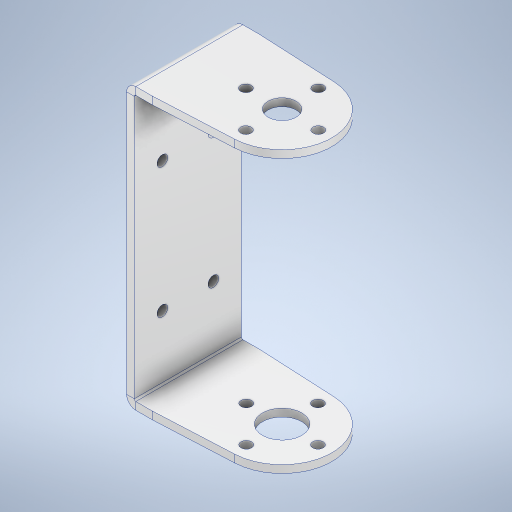
# Autodesk Inventor part: ㄷ_frame_2
Saved by Autodesk Inventor 2023 (Build 270158000, 158)
## iProperties
Created: 2022-10-22
Part Number: ㄷ_frame_2
Material: Aluminum 6061
Document SubType Name: Sheet Metal
Designer: chanh
Density: 2.7 g/cm^3
Sheet Metal Rule: Default_mm
Appearance: Aluminum - Flat
Flat Pattern Width: 2.1 cm
Flat Pattern Length: 10.9059 cm
Flat Pattern Area: 22.9023 cm^2
Sheet Metal Width: 21.000 mm
Sheet Metal Length: 109.059 mm
Sheet Metal Area: 2290.230 mm^2
품번: 20
Author: chanh
Autodesk Inventor part; units mm, degrees
ref_plane "YZ Plane" through (0, 0, 0) normal (1, 0, 0) x (0, 1, 0)
ref_plane "Work Plane1" through (34.2931, 25.9114, -33.2342) normal (0, 1, 0) x (-1, 0, 0)
sketch "Sketch2" plane through (34.2931, 25.9114, -33.2342) normal (0, 1, 0) x (-1, 0, 0)
  circle A0 centre (9.75, 7.1) radius 0.7835
  circle A1 centre (16.85, 0) radius 0.7835
  circle A2 centre (9.75, -7.1) radius 0.7835
  circle A3 centre (2.65, 0) radius 0.7835
  circle A4 centre (4.7295, -5.0205) radius 0.7835
  circle A5 centre (14.7705, -5.0205) radius 0.7835
  circle A6 centre (14.7705, 5.0205) radius 0.7835
  circle A7 centre (4.7295, 5.0205) radius 0.7835
  circle A8 centre (9.75, 0) radius 3.8
  circle A9 centre (9.75, 0) radius 9.75
  circle A10 centre (9.75, 0) radius 2.75
  line L0 (29.75, -10.5) -> (29.75, 10.5)
  line L1 (29.75, -10.5) -> (24.75, -10.5)
  line L2 (29.75, 10.5) -> (24.75, 10.5)
  line L3 (24.75, -10.5) -> (9.2707, -9.7382)
  line L4 (24.75, 10.5) -> (9.2707, 9.7382)
  circle A11 centre (9.75, -7.1) radius 1.05
  circle A12 centre (16.85, 0) radius 1.05
  circle A13 centre (9.75, 7.1) radius 1.05
  circle A14 centre (2.65, 0) radius 1.05
  point P0 (34.2931, 33.2342)
  point P1 (29.75, 0)
  dimension "d2" = 5.5
  dimension "d4" = 21
  dimension "d5" = 5
  dimension "d6" = 20
  dimension "d36" = 2.1
  measures "d2" diameter of A10
  measures "d4" distance of L0.start L0.end
  measures "d5" distance of L0.start L1.end
  measures "d6" distance from line of A8.centre L0
  measures "d36" diameter of A11
extrude "Plate2" add sketch "Sketch2" along normal blind 1.5 contours A4 | A5 | A6 | A7 | A8 | A9 | A9 L4 L2 L0 L1 L3
sketch "Sketch3" plane through (6.0431, 27.4114, -43.7342) normal (-1, 0, 0) x (0, -1, 0)
  line L0 (0, 21) -> (0, 0)
  line L1 (0, 0) -> (55, 0)
  line L2 (55, 0) -> (55, 21)
  line L3 (55, 21) -> (0, 21)
  constraints: 6 end point, 1 horizontal, 1 perpendicular, 1 vertical
edge flange "Flange1" height 55 angle 90 thickness 1.5 bend radius 0.31 thickness toward (-1, 0, 0) relief tear relief width 1.5 relief depth 0.75 edges at (4.5431, 25.9114, -33.2342) wall of the first edge with corners at (6.0431, 27.4114, -22.7342) (6.0431, 27.4114, -43.7342) (6.0431, -27.5886, -43.7342) (6.0431, -27.5886, -22.7342)
bend "Bend1"
corner "Corner1"
sketch "Sketch4" plane through (4.5431, -26.0886, -43.7342) normal (0, -1, 0) x (1, 0, 0)
  line L0 (0, 21) -> (0, 0)
  line L1 (0, 0) -> (30, 0)
  line L2 (30, 0) -> (30, 21)
  line L3 (30, 21) -> (0, 21)
  constraints: 6 end point, 1 horizontal, 1 perpendicular, 1 vertical
edge flange "Flange2" height 30 angle 90 thickness 1.5 bend radius 0.31 thickness toward (0, -1, 0) relief tear relief width 1.5 relief depth 0.75 edges at (6.0431, -27.5886, -33.2342) wall of the first edge with corners at (4.5431, -26.0886, -22.7342) (4.5431, -26.0886, -43.7342) (34.5431, -26.0886, -43.7342) (34.5431, -26.0886, -22.7342)
bend "Bend2"
corner "Corner2"
sketch "Sketch5" plane through (34.5431, -27.5886, -43.7342) normal (0, -1, 0) x (1, 0, 0)
  circle A0 centre (-10, 10.5) radius 3.8 projected
  circle A1 centre (-10, 10.5) radius 3.85
  point P0 (-34.5431, 43.7342)
  dimension "d37" = 7.7
  constraints: 1 centre point, 1 coincident
  measures "d37" diameter of A1
extrude "Cut1" cut sketch "Sketch5" against normal blind 1.5 contours A0 | A1
sketch "Sketch6" plane through (34.5431, -27.5886, -43.7342) normal (0, -1, 0) x (1, 0, 0)
  circle A0 centre (-10, 17.525) radius 0.7835 projected
  circle A1 centre (-2.975, 10.5) radius 0.7835 projected
  circle A2 centre (-10, 3.475) radius 0.7835 projected
  circle A3 centre (-17.025, 10.5) radius 0.7835 projected
  circle A4 centre (-10, 10.5) radius 9.75 projected
  line L0 (-25, 21) -> (-9.5207, 20.2382) projected
  line L1 (-9.5207, 0.7618) -> (-25, 0) projected
  line L2 (-28.19, 21) -> (0, 21) projected
  line L3 (0, 21) -> (0, 0) projected
  line L4 (0, 0) -> (-28.19, 0) projected
  line L5 (-28.19, 21) -> (-30, 21) projected
  line L6 (-30, 0) -> (-28.19, 0) projected
  circle A5 centre (-2.975, 10.5) radius 1.05
  circle A6 centre (-10, 17.525) radius 1.05
  circle A7 centre (-17.025, 10.5) radius 1.05
  circle A8 centre (-10, 3.475) radius 1.05
  point P0 (-34.5431, 43.7342)
  dimension "d35" = 2.1
  constraints: 4 centre point, 4 coincident, 3 equal radius
  measures "d35" diameter of A5
extrude "Cut2" cut sketch "Sketch6" against normal blind 1.5 contours A0 | A1 | A2 | A3 | A4 L0 L2 L3 L4 L1 | A5 | A6 | A7 | A8
ref_plane "작업 평면2" through (4.5431, 25.6014, -33.2342) normal (0, 0, 1) x (1, 0, 0)
sketch "Sketch7" plane through (6.0431, 25.6014, -22.7342) normal (1, 0, 0) x (0, 0, -1)
  circle A0 centre (5.5, -13.69) radius 0.7835 projected
  circle A1 centre (15.5, -13.69) radius 0.7835 projected
  circle A2 centre (5.5, -39.19) radius 0.7835 projected
  circle A3 centre (15.5, -39.19) radius 0.7835 projected
  circle A4 centre (5.5, -13.69) radius 1.05
  circle A5 centre (15.5, -13.69) radius 1.05
  circle A6 centre (5.5, -39.19) radius 1.05
  circle A7 centre (15.5, -39.19) radius 1.05
  point P0 (-22.7342, -25.6014)
  dimension "d34" = 2.1
  constraints: 4 centre point, 4 coincident, 3 equal radius
  measures "d34" diameter of A4
extrude "Cut3" cut sketch "Sketch7" against normal blind 1.5 contours A0 | A1 | A2 | A3 | A4 | A5 | A6 | A7
equation "\"d28\" = Thickness"
equation "\"d30\" = Thickness"
equation "\"d32\" = Thickness"
equation "\"d7\" = Thickness"
equation "\"d8\" = BendReliefWidth"
equation "\"d9\" = BendReliefDepth"
equation "\"d10\" = MinimumRemnant"
equation "\"d11\" = TransitionRadius"
equation "\"d14\" = BendRadius"
equation "\"d15\" = CornerReliefSize"
equation "\"d16\" = GapSize"
equation "\"d17\" = JacobiRadiusSize"
equation "\"d18\" = BendReliefWidth"
equation "\"d19\" = BendReliefDepth"
equation "\"d20\" = MinimumRemnant"
equation "\"d21\" = TransitionRadius"
equation "\"d24\" = BendRadius"
equation "\"d25\" = CornerReliefSize"
equation "\"d26\" = GapSize"
equation "\"d27\" = JacobiRadiusSize"
equation "\"BendReliefWidth\" = Thickness"
equation "\"BendReliefDepth\" = 0.5 * Thickness"
equation "\"CornerReliefSize\" = 4 * Thickness"
equation "\"MinimumRemnant\" = 2 * Thickness"
equation "\"TransitionRadius\" = BendRadius"
equation "\"JacobiRadiusSize\" = BendRadius"
equation "\"GapSize\" = Thickness"
equation "\"Thickness\" = 1.5"
equation "\"BendRadius\" = 0.31"
body "Solid2"
